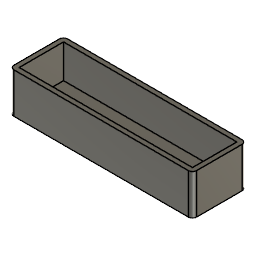
boody (Autodesk Fusion 360 design; units mm, degrees)
part number: 2026-01-20-21-01-43-835
Autodesk Fusion 360 part; units mm, degrees
sketch "Sketch1" plane through (0, 0, 0) normal (0, 0, 1) x (1, 0, 0)
  line L0 (0, 0) -> (136, 0)
  line L1 (136, 0) -> (136, 40)
  line L2 (136, 40) -> (0, 40)
  line L3 (0, 40) -> (0, 0)
  line L4 (3.5, 36.5) -> (132.5, 36.5)
  line L5 (132.5, 36.5) -> (132.5, 3.5)
  line L6 (132.5, 3.5) -> (3.5, 3.5)
  line L7 (3.5, 3.5) -> (3.5, 36.5)
  line L8 (62.8, 7.5) -> (72.3, 7.5)
  line L9 (72.3, 7.5) -> (72.3, 3.5)
  line L10 (72.3, 3.5) -> (62.8, 3.5)
  line L11 (62.8, 3.5) -> (62.8, 7.5)
  dimension "d1" = 40
  dimension "d2" = 136
  dimension "d3" = 129
  dimension "d4" = 33
  dimension "d5" = 3.5
  dimension "d6" = 3.5
  dimension "d7" = 4
  dimension "d8" = 9.5
  dimension "d9" = 59.3
  constraint horizontal L0
  constraint vertical L1
  constraint horizontal L2
  constraint vertical L3
  constraint coincident L0.start L3.end
  constraint horizontal L4
  constraint vertical L5
  constraint horizontal L6
  constraint vertical L7
  constraint horizontal L8
  constraint vertical L9
  constraint horizontal L10
  constraint vertical L11
  constraint coincident L6 L9.end
  measures "d1" distance of L0.start L2.end
  measures "d2" distance of L0.start L0.end
  measures "d3" distance of L5.end L6.end
  measures "d4" distance of L4.end L5.end
  measures "d5" distance of L1 L5
  measures "d6" distance of L0 L6
  measures "d7" distance of L8.start L10.end
  measures "d8" distance of L9.end L10.end
  measures "d9" distance of L7 L11
extrude "Extrude1" add sketch "Sketch1" along normal blind 5 contours L4 L5 L6 L7 L8 L9 L11 makes body 1
extrude "Extrude2" add sketch "Sketch1" along normal blind 30 separate body makes body 2
fillet "Fillet1" radius 3 4 edges at (0, 0, 15) (136, 0, 15) (136, 40, 15) (0, 40, 15) on bodies 2
